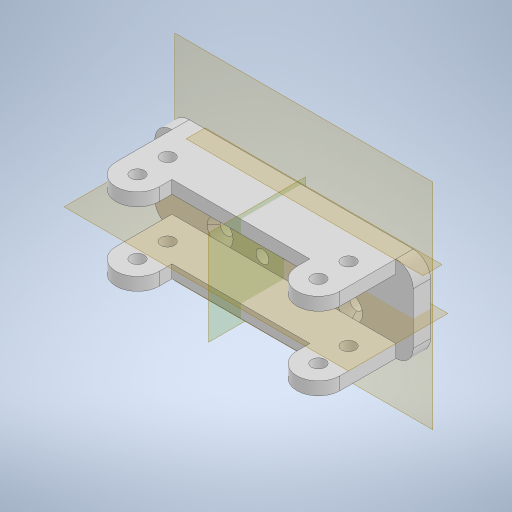
# Autodesk Inventor part: крепление_кракаса
Saved by Autodesk Inventor 2023.1 (Build 271208000, 208)
## iProperties
Created: 2025-09-24
Part Number: крепление_кракаса
Material: Типовые
Document SubType Name: Modeling
Designer: DELL
Density: 1 g/cm^3
Appearance: По умолчанию
Author: DELL
Autodesk Inventor part; units mm, degrees
ref_plane "YZ Plane" through (0, 0, 0) normal (1, 0, 0) x (0, 1, 0)
ref_plane "XZ Plane" through (0, 0, 0) normal (0, 1, 0) x (-1, 0, 0)
ref_plane "XY Plane" through (0, 0, 0) normal (0, 0, 1) x (1, 0, 0)
ref_plane "РабПлоскость1" through (0, 0, 0) normal (0, 0, 1) x (1, 0, 0)
sketch "Эскиз1" plane through (0, 0, 0) normal (0, 0, 1) x (1, 0, 0)
  ellipse E0 centre (9.7167, 5.0001) end of major axis (8.2166, 5.0001) minor radius 1.5001
  circle A0 centre (9.7169, 14.9999) radius 1.5003
  circle A1 centre (19.3814, 15) radius 1.5
  circle A2 centre (19.5198, 5) radius 1.5
  ellipse E1 centre (29.5544, 5.0002) end of major axis (28.1004, 5.3695) minor radius 1.5002
  circle A3 centre (29.5547, 15.0004) radius 1.5006
  circle A4 centre (39.7965, 14.9999) radius 1.4999
  ellipse E2 centre (39.7967, 5) end of major axis (39.8584, 3.5011) minor radius 1.5002
  circle A5 centre (24.5262, 10.0003) radius 3.0726
  line L0 (-1.4738, 20.0003) -> (50.5262, 20.0003)
  line L1 (54.5262, 16.0003) -> (54.5262, 4.0003)
  line L2 (50.5262, 0.0003) -> (-1.4738, 0.0003)
  line L3 (-5.4738, 4.0003) -> (-5.4738, 16.0003)
  line L4 (-5.4738, 20.0003) -> (54.5262, 0.0003) construction
  line L5 (54.5262, 20.0003) -> (-5.4738, 0.0003) construction
  arc A6 (54.5262, 16.0003) -> (50.5262, 20.0003) centre (50.5262, 16.0003) ccw
  arc A7 (50.5262, 0.0003) -> (54.5262, 4.0003) centre (50.5262, 4.0003) ccw
  arc A8 (-1.4738, 20.0003) -> (-5.4738, 16.0003) centre (-1.4738, 16.0003) ccw
  arc A9 (-5.4738, 4.0003) -> (-1.4738, 0.0003) centre (-1.4738, 4.0003) ccw
  dimension "d0" = 60
  dimension "d1" = 20
  dimension "d2" = 4
  constraints: 12 end point, 11 centre point, 8 point on circle, 8 point on line, 8 tangent, 3 equal radius, 2 midpoint, 2 parallel, 1 horizontal, 1 perpendicular, 4 other
  measures "d0" distance of L4.start L5.start
  measures "d1" distance of L5.start L4.end
  measures "d2" radius of A6
extrude "Выдавливание1" add sketch "Эскиз1" along normal blind 4
chamfer "Фаска1" distance 1.5 angle 45 8 edges at (8.2166, 14.9999, 4) (39.735, 6.4989, 4) (38.2966, 14.9999, 4) (11.2168, 5.0001, 4) (18.0198, 5, 0) (17.8814, 15, 0) (28.0542, 15.0004, 0) (31.0085, 4.6309, 0)
ref_plane "РабПлоскость2" through (50.5262, 20.0003, 0) normal (0, 1, 0) x (-1, 0, 0)
sketch "Эскиз2" plane through (50.5262, 20.0003, 0) normal (0, 1, 0) x (-1, 0, 0)
  line L0 (0, 0) -> (52, 0) construction
  line L1 (52, 0) -> (52, 4) construction
  line L2 (0, 4) -> (52, 4) construction
  line L3 (0, 0) -> (0, 4) construction
  line L4 (0, 0) -> (0, 4) projected
  line L5 (52, 4) -> (0, 4) projected
  line L6 (0, 0) -> (10, 0)
  line L7 (10, 0) -> (10, 4)
  line L8 (10, 4) -> (0, 4)
  line L9 (0, 4) -> (0, 0)
  circle A0 centre (5, 10) radius 1.6
  circle A1 centre (5, 10) radius 5
  line L10 (0, 4) -> (-4, 4) projected
  line L11 (0, 10) -> (0, 4)
  line L12 (10, 10) -> (10, 4)
  circle A2 centre (5, 17) radius 1.6
  circle A3 centre (5, 17) radius 5
  line L13 (5, 10) -> (5, 17)
  line L14 (0, 10) -> (0, 17)
  line L15 (10, 17) -> (10, 10)
  point P0 (8.7764, 20.2771)
  dimension "d8" = 10
  dimension "d9" = 3.2
  dimension "d10" = 3.2
  dimension "d11" = 10
  dimension "d12" = 10
  dimension "d13" = 7
  dimension "d14" = 6
  constraints: 18 end point, 5 point on circle, 4 centre point, 3 coincident, 3 vertical, 2 parallel, 1 horizontal, 1 perpendicular, 1 point on line, 1 tangent
  measures "d8" distance of L8.end L7.end
  measures "d9" diameter of A0
  measures "d10" diameter of A2
  measures "d11" diameter of A1
  measures "d12" diameter of A3
  measures "d13" distance of L13.start L13.end
  measures "d14" distance of L12.start L7.end
extrude "Выдавливание2" add sketch "Эскиз2" against normal blind 3 contours L11 A1 L12 L5 | A1 A3 | L14 A3 A1 | A1 A3 L15 | A3 A1 | A1 L13 A3 | A3 L13 A1
ref_plane "РабПлоскость3" through (-1.4738, 10.0003, 0) normal (0, 1, 0) x (1, 0, 0)
mirror "Зеркальное отражение1" about plane through (-1.4738, 10.0003, 0) normal (0, 1, 0) of "Выдавливание2"
ref_plane "РабПлоскость4" through (24.5262, 4.0003, 0) normal (-1, 0, 0) x (0, 0, 1)
mirror "Зеркальное отражение2" about plane through (24.5262, 4.0003, 0) normal (-1, 0, 0) of "Выдавливание2", "Зеркальное отражение1"
sketch "Эскиз3" plane through (0, 0, 4) normal (0, 0, 1) x (1, 0, 0)
  line L0 (40.5262, 20.0003) -> (8.5262, 20.0003) projected
  line L1 (40.5262, 17.0003) -> (8.5262, 17.0003)
  line L2 (8.5262, 17.0003) -> (8.5262, 20.0003)
  line L3 (8.5262, 20.0003) -> (40.5262, 20.0003)
  line L4 (40.5262, 20.0003) -> (40.5262, 17.0003)
  line L5 (40.5262, 17.0003) -> (8.5262, 20.0003) construction
  line L6 (8.5262, 17.0003) -> (40.5262, 20.0003) construction
  line L7 (8.5262, 20.0003) -> (8.5262, 17.0003) projected
  line L8 (8.5262, 0.0003) -> (40.5262, 0.0003)
  line L9 (40.5262, 0.0003) -> (40.5262, 3.0003)
  line L10 (40.5262, 3.0003) -> (8.5262, 3.0003)
  line L11 (8.5262, 3.0003) -> (8.5262, 0.0003)
  line L12 (8.5262, 0.0003) -> (40.5262, 3.0003) construction
  line L13 (40.5262, 0.0003) -> (8.5262, 3.0003) construction
  line L14 (40.5262, 0.0003) -> (40.5262, 3.0003) projected
  line L15 (8.5262, 0.0003) -> (40.5262, 0.0003) projected
  point P0 (0, 0)
  point P1 (24.5262, 18.5003)
  point P2 (8.5262, 18.5003)
  point P3 (40.5262, 20.0003)
  point P4 (24.5262, 1.5003)
  point P5 (40.5262, 1.5003)
  point P6 (24.5262, 0.0003)
  dimension "d22" = 32
  dimension "d23" = 3
  dimension "d27" = 32
  dimension "d28" = 3
  constraints: 24 end point, 10 midpoint, 4 parallel, 2 horizontal, 2 perpendicular, 1 point on line
  measures "d22" distance of L1.start L1.end
  measures "d23" distance between parallel lines of L0 L1
  measures "d27" distance of L10.end L9.end
  measures "d28" distance of L9.end L8.end
extrude "Выдавливание3" add sketch "Эскиз3" along normal blind 10
